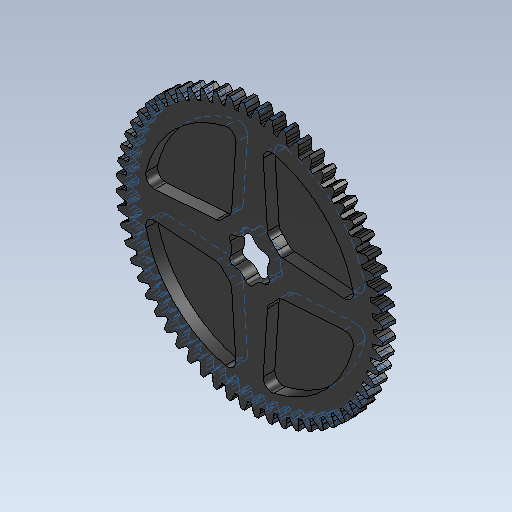
# Autodesk Inventor part: m1z60
Saved by Autodesk Inventor 2020 (Build 240168000, 168)
## iProperties
Created: 2020-10-28
Part Number: m1z60
Material: ポリカーボネート、クリア
Document SubType Name: Modeling
Designer: AA19065
Density: 1.2 g/cm^3
Appearance: 光沢 - 黒
Mass: 5.9358 g
Surface Area: 74.7819 cm^2
Volume: 4.9465 cm^3
Author: AA19065
Autodesk Inventor part; units mm, degrees
(part 1 of 2)
ref_plane "YZ Plane" through (0, 0, 0) normal (1, 0, 0) x (0, 1, 0)
ref_plane "XZ Plane" through (0, 0, 0) normal (0, 1, 0) x (-1, 0, 0)
ref_plane "XY Plane" through (0, 0, 0) normal (0, 0, 1) x (1, 0, 0)
sketch "スケッチ1" plane through (0, 0, 0) normal (0, 0, 1) x (1, 0, 0)
  arc A0 (149.0364, 134.2758) -> (148.8992, 133.7472) centre (155.551, 132.3028) ccw
  arc A1 (149.2947, 135.0135) -> (149.0364, 134.2758) centre (157.799, 131.622) ccw
  arc A2 (149.73, 135.9756) -> (149.2947, 135.0135) centre (160.0948, 130.7064) ccw
  arc A3 (145.9733, 134.1715) -> (145.8921, 133.6315) centre (152.6585, 132.8903) ccw
  arc A4 (146.1531, 134.9321) -> (145.9733, 134.1715) centre (154.9653, 132.4481) ccw
  arc A5 (146.4854, 135.9345) -> (146.1531, 134.9321) centre (157.3443, 131.7776) ccw
  arc A6 (142.9379, 133.7476) -> (142.9136, 133.202) centre (149.7204, 133.1722) ccw
  arc A7 (143.0372, 134.5228) -> (142.9379, 133.7476) centre (152.0608, 132.9736) ccw
  arc A8 (143.2629, 135.5544) -> (143.0372, 134.5228) centre (154.4968, 132.5553) ccw
  arc A9 (139.9634, 133.0087) -> (139.9963, 132.4636) centre (146.7689, 133.1454) ccw
  arc A10 (139.9811, 133.7901) -> (139.9634, 133.0087) centre (149.1173, 133.1925) ccw
  arc A11 (140.0978, 134.8396) -> (139.9811, 133.7901) centre (151.5836, 133.0312) ccw
  arc A12 (137.0825, 131.963) -> (137.1722, 131.4243) centre (143.8364, 132.8103) ccw
  arc A13 (137.0184, 132.7419) -> (137.0825, 131.963) centre (146.167, 133.1026) ccw
  arc A14 (137.0248, 133.7979) -> (137.0184, 132.7419) centre (148.6367, 133.2) ccw
  arc A15 (134.3267, 130.6218) -> (134.4721, 130.0954) centre (140.955, 132.1704) ccw
  arc A16 (134.1815, 131.3898) -> (134.3267, 130.6218) centre (143.2422, 132.7048) ccw
  arc A17 (134.0774, 132.4406) -> (134.1815, 131.3898) centre (145.6882, 133.0598) ccw
  arc A18 (131.7261, 128.9999) -> (131.9258, 128.4916) centre (138.1562, 131.2329) ccw
  arc A19 (131.5014, 129.7485) -> (131.7261, 128.9999) centre (140.3751, 132.0034) ccw
  arc A20 (131.2881, 130.7827) -> (131.5014, 129.7485) centre (142.7706, 132.6122) ccw
  arc A21 (129.3093, 127.1151) -> (129.561, 126.6305) centre (135.4708, 130.008) ccw
  arc A22 (129.0076, 127.8361) -> (129.3093, 127.1151) centre (137.597, 131.0062) ccw
  arc A23 (128.6874, 128.8424) -> (129.0076, 127.8361) centre (139.9157, 131.862) ccw
  arc A24 (127.1028, 124.988) -> (127.4038, 124.5323) centre (132.9281, 128.5091) ccw
  arc A25 (126.7274, 125.6735) -> (127.1028, 124.988) centre (134.9383, 129.7241) ccw
  arc A26 (126.3037, 126.6408) -> (126.7274, 125.6735) centre (137.1549, 130.8176) ccw
  arc A27 (125.1307, 122.6419) -> (125.4777, 122.2202) centre (130.5561, 126.7526) ccw
  arc A28 (124.6857, 123.2844) -> (125.1307, 122.6419) centre (132.4282, 128.1711) ccw
  arc A29 (124.1632, 124.2021) -> (124.6857, 123.2844) centre (134.5184, 129.4903) ccw
  arc A30 (123.4146, 120.1025) -> (123.8038, 119.7193) centre (128.3806, 124.7578) ccw
  arc A31 (122.9049, 120.695) -> (123.4146, 120.1025) centre (130.0942, 126.3642) ccw
  arc A32 (122.2894, 121.553) -> (122.9049, 120.695) centre (132.035, 127.8946) ccw
  arc A33 (121.9734, 117.3976) -> (122.4005, 117.0573) centre (126.4256, 122.5465) ccw
  arc A34 (121.4046, 117.9336) -> (121.9734, 117.3976) centre (127.9619, 124.3232) ccw
  arc A35 (120.7027, 118.7226) -> (121.4046, 117.9336) centre (129.7321, 126.0481) ccw
  arc A36 (120.8228, 114.5569) -> (121.2831, 114.2631) centre (124.7124, 120.143) ccw
  arc A37 (120.2011, 115.0305) -> (120.8228, 114.5569) centre (126.0546, 122.0705) ccw
  arc A38 (119.4206, 115.7418) -> (120.2011, 115.0305) centre (127.6348, 123.9711) ccw
  arc A39 (119.9755, 111.6115) -> (120.464, 111.3674) centre (123.2598, 117.5735) ccw
  arc A40 (119.3076, 112.0175) -> (119.9755, 111.6115) centre (124.3932, 119.6308) ccw
  arc A41 (118.457, 112.6433) -> (119.3076, 112.0175) centre (125.7661, 121.6861) ccw
  arc A42 (119.4406, 108.5937) -> (119.952, 108.4019) centre (122.0838, 114.8663) ccw
  arc A43 (118.734, 108.9276) -> (119.4406, 108.5937) centre (122.9959, 117.0308) ccw
  arc A44 (117.8227, 109.4611) -> (118.734, 108.9276) centre (124.1464, 119.2184) ccw
  arc A45 (119.2242, 105.5364) -> (119.7528, 105.3992) centre (121.1972, 112.051) ccw
  arc A46 (118.4865, 105.7947) -> (119.2242, 105.5364) centre (121.878, 114.299) ccw
  arc A47 (117.5244, 106.23) -> (118.4865, 105.7947) centre (122.7936, 116.5948) ccw
  arc A48 (119.3285, 102.4733) -> (119.8685, 102.3921) centre (120.6097, 109.1585) ccw
  arc A49 (118.5679, 102.6531) -> (119.3285, 102.4733) centre (121.0519, 111.4653) ccw
  arc A50 (117.5655, 102.9854) -> (118.5679, 102.6531) centre (121.7224, 113.8443) ccw
  arc A51 (119.7524, 99.4379) -> (120.298, 99.4136) centre (120.3278, 106.2204) ccw
  arc A52 (118.9772, 99.5372) -> (119.7524, 99.4379) centre (120.5264, 108.5608) ccw
  arc A53 (117.9456, 99.7629) -> (118.9772, 99.5372) centre (120.9447, 110.9968) ccw
  arc A54 (120.4913, 96.4634) -> (121.0364, 96.4963) centre (120.3546, 103.2689) ccw
  arc A55 (119.7099, 96.4811) -> (120.4913, 96.4634) centre (120.3075, 105.6173) ccw
  arc A56 (118.6604, 96.5978) -> (119.7099, 96.4811) centre (120.4688, 108.0836) ccw
  arc A57 (121.537, 93.5825) -> (122.0757, 93.6722) centre (120.6897, 100.3364) ccw
  arc A58 (120.7581, 93.5184) -> (121.537, 93.5825) centre (120.3974, 102.667) ccw
  arc A59 (119.7021, 93.5248) -> (120.7581, 93.5184) centre (120.3, 105.1367) ccw
  arc A60 (122.8782, 90.8267) -> (123.4046, 90.9721) centre (121.3296, 97.455) ccw
  arc A61 (122.1102, 90.6815) -> (122.8782, 90.8267) centre (120.7952, 99.7422) ccw
  arc A62 (121.0594, 90.5774) -> (122.1102, 90.6815) centre (120.4402, 102.1882) ccw
  arc A63 (124.5001, 88.2261) -> (125.0084, 88.4258) centre (122.2671, 94.6562) ccw
  arc A64 (123.7515, 88.0014) -> (124.5001, 88.2261) centre (121.4966, 96.8751) ccw
  arc A65 (122.7173, 87.7881) -> (123.7515, 88.0014) centre (120.8878, 99.2706) ccw
  arc A66 (126.3849, 85.8093) -> (126.8695, 86.061) centre (123.492, 91.9708) ccw
  arc A67 (125.6639, 85.5076) -> (126.3849, 85.8093) centre (122.4938, 94.097) ccw
  arc A68 (124.6576, 85.1874) -> (125.6639, 85.5076) centre (121.638, 96.4157) ccw
  arc A69 (128.512, 83.6028) -> (128.9677, 83.9038) centre (124.9909, 89.4281) ccw
  arc A70 (127.8265, 83.2274) -> (128.512, 83.6028) centre (123.7759, 91.4383) ccw
  arc A71 (126.8592, 82.8037) -> (127.8265, 83.2274) centre (122.6824, 93.6549) ccw
  arc A72 (130.8581, 81.6307) -> (131.2798, 81.9777) centre (126.7474, 87.0561) ccw
  arc A73 (130.2156, 81.1857) -> (130.8581, 81.6307) centre (125.3289, 88.9282) ccw
  arc A74 (129.2979, 80.6632) -> (130.2156, 81.1857) centre (124.0097, 91.0184) ccw
  arc A75 (133.3975, 79.9146) -> (133.7807, 80.3038) centre (128.7422, 84.8806) ccw
  arc A76 (132.805, 79.4049) -> (133.3975, 79.9146) centre (127.1358, 86.5942) ccw
  arc A77 (131.947, 78.7894) -> (132.805, 79.4049) centre (125.6054, 88.535) ccw
  arc A78 (136.1024, 78.4734) -> (136.4427, 78.9005) centre (130.9535, 82.9256) ccw
  arc A79 (135.5664, 77.9046) -> (136.1024, 78.4734) centre (129.1768, 84.4619) ccw
  arc A80 (134.7774, 77.2027) -> (135.5664, 77.9046) centre (127.4519, 86.2321) ccw
  arc A81 (138.9431, 77.3228) -> (139.2369, 77.7831) centre (133.357, 81.2124) ccw
  arc A82 (138.4695, 76.7011) -> (138.9431, 77.3228) centre (131.4295, 82.5546) ccw
  arc A83 (137.7582, 75.9206) -> (138.4695, 76.7011) centre (129.529, 84.1348) ccw
  arc A84 (141.8885, 76.4755) -> (142.1326, 76.964) centre (135.9265, 79.7598) ccw
  arc A85 (141.4825, 75.8076) -> (141.8885, 76.4755) centre (133.8692, 80.8932) ccw
  arc A86 (140.8567, 74.957) -> (141.4825, 75.8076) centre (131.8139, 82.2661) ccw
  arc A87 (144.9063, 75.9406) -> (145.0981, 76.452) centre (138.6337, 78.5838) ccw
  arc A88 (144.5724, 75.234) -> (144.9063, 75.9406) centre (136.4692, 79.4959) ccw
  arc A89 (144.0389, 74.3227) -> (144.5724, 75.234) centre (134.2816, 80.6464) ccw
  arc A90 (147.9636, 75.7242) -> (148.1008, 76.2528) centre (141.449, 77.6972) ccw
  arc A91 (147.7053, 74.9865) -> (147.9636, 75.7242) centre (139.201, 78.378) ccw
  arc A92 (147.27, 74.0244) -> (147.7053, 74.9865) centre (136.9052, 79.2936) ccw
  arc A93 (151.0267, 75.8285) -> (151.1079, 76.3685) centre (144.3415, 77.1097) ccw
  arc A94 (150.8469, 75.0679) -> (151.0267, 75.8285) centre (142.0347, 77.5519) ccw
  arc A95 (150.5146, 74.0655) -> (150.8469, 75.0679) centre (139.6557, 78.2224) ccw
  arc A96 (154.0621, 76.2524) -> (154.0864, 76.798) centre (147.2796, 76.8278) ccw
  arc A97 (153.9628, 75.4772) -> (154.0621, 76.2524) centre (144.9392, 77.0264) ccw
  arc A98 (153.7371, 74.4456) -> (153.9628, 75.4772) centre (142.5032, 77.4447) ccw
  arc A99 (157.0366, 76.9913) -> (157.0037, 77.5364) centre (150.2311, 76.8546) ccw
  arc A100 (157.0189, 76.2099) -> (157.0366, 76.9913) centre (147.8827, 76.8075) ccw
  arc A101 (156.9022, 75.1604) -> (157.0189, 76.2099) centre (145.4164, 76.9688) ccw
  arc A102 (159.9175, 78.037) -> (159.8278, 78.5757) centre (153.1636, 77.1897) ccw
  arc A103 (159.9816, 77.2581) -> (159.9175, 78.037) centre (150.833, 76.8974) ccw
  arc A104 (159.9752, 76.2021) -> (159.9816, 77.2581) centre (148.3633, 76.8) ccw
  arc A105 (162.6733, 79.3782) -> (162.5279, 79.9046) centre (156.045, 77.8296) ccw
  arc A106 (162.8185, 78.6102) -> (162.6733, 79.3782) centre (153.7578, 77.2952) ccw
  arc A107 (162.9226, 77.5594) -> (162.8185, 78.6102) centre (151.3118, 76.9402) ccw
  arc A108 (165.2739, 81.0001) -> (165.0742, 81.5084) centre (158.8438, 78.7671) ccw
  arc A109 (165.4986, 80.2515) -> (165.2739, 81.0001) centre (156.6249, 77.9966) ccw
  arc A110 (165.7119, 79.2173) -> (165.4986, 80.2515) centre (154.2294, 77.3878) ccw
  arc A111 (167.6907, 82.8849) -> (167.439, 83.3695) centre (161.5292, 79.992) ccw
  arc A112 (167.9924, 82.1639) -> (167.6907, 82.8849) centre (159.403, 78.9938) ccw
  arc A113 (168.3126, 81.1576) -> (167.9924, 82.1639) centre (157.0843, 78.138) ccw
  arc A114 (169.8972, 85.012) -> (169.5962, 85.4677) centre (164.0719, 81.4909) ccw
  arc A115 (170.2726, 84.3265) -> (169.8972, 85.012) centre (162.0617, 80.2759) ccw
  arc A116 (170.6963, 83.3592) -> (170.2726, 84.3265) centre (159.8451, 79.1824) ccw
  arc A117 (171.8693, 87.3581) -> (171.5223, 87.7798) centre (166.4439, 83.2474) ccw
  arc A118 (172.3143, 86.7156) -> (171.8693, 87.3581) centre (164.5718, 81.8289) ccw
  arc A119 (172.8368, 85.7979) -> (172.3143, 86.7156) centre (162.4816, 80.5097) ccw
  arc A120 (173.5854, 89.8975) -> (173.1962, 90.2807) centre (168.6194, 85.2422) ccw
  arc A121 (174.0951, 89.305) -> (173.5854, 89.8975) centre (166.9058, 83.6358) ccw
  arc A122 (174.7106, 88.447) -> (174.0951, 89.305) centre (164.965, 82.1054) ccw
  arc A123 (175.0266, 92.6024) -> (174.5995, 92.9427) centre (170.5744, 87.4535) ccw
  arc A124 (175.5954, 92.0664) -> (175.0266, 92.6024) centre (169.0381, 85.6768) ccw
  arc A125 (176.2973, 91.2774) -> (175.5954, 92.0664) centre (167.2679, 83.9519) ccw
  arc A126 (176.1772, 95.4431) -> (175.7169, 95.7369) centre (172.2876, 89.857) ccw
  arc A127 (176.7989, 94.9695) -> (176.1772, 95.4431) centre (170.9454, 87.9295) ccw
  arc A128 (177.5794, 94.2582) -> (176.7989, 94.9695) centre (169.3652, 86.029) ccw
  arc A129 (177.0245, 98.3885) -> (176.536, 98.6326) centre (173.7402, 92.4265) ccw
  arc A130 (177.6924, 97.9825) -> (177.0245, 98.3885) centre (172.6068, 90.3692) ccw
  arc A131 (178.543, 97.3567) -> (177.6924, 97.9825) centre (171.2339, 88.3139) ccw
  arc A132 (177.5594, 101.4063) -> (177.048, 101.5981) centre (174.9162, 95.1337) ccw
  arc A133 (178.266, 101.0724) -> (177.5594, 101.4063) centre (174.0041, 92.9692) ccw
  arc A134 (179.1773, 100.5389) -> (178.266, 101.0724) centre (172.8536, 90.7816) ccw
  arc A135 (177.7758, 104.4636) -> (177.2472, 104.6008) centre (175.8028, 97.949) ccw
  arc A136 (178.5135, 104.2053) -> (177.7758, 104.4636) centre (175.122, 95.701) ccw
  arc A137 (179.4756, 103.77) -> (178.5135, 104.2053) centre (174.2064, 93.4052) ccw
  arc A138 (177.6715, 107.5267) -> (177.1315, 107.6079) centre (176.3903, 100.8415) ccw
  arc A139 (178.4321, 107.3469) -> (177.6715, 107.5267) centre (175.9481, 98.5347) ccw
  arc A140 (179.4345, 107.0146) -> (178.4321, 107.3469) centre (175.2776, 96.1557) ccw
  arc A141 (177.2476, 110.5621) -> (176.702, 110.5864) centre (176.6722, 103.7796) ccw
  arc A142 (178.0228, 110.4628) -> (177.2476, 110.5621) centre (176.4736, 101.4392) ccw
  arc A143 (179.0544, 110.2371) -> (178.0228, 110.4628) centre (176.0553, 99.0032) ccw
  arc A144 (176.5087, 113.5366) -> (175.9636, 113.5037) centre (176.6454, 106.7311) ccw
  arc A145 (177.2901, 113.5189) -> (176.5087, 113.5366) centre (176.6925, 104.3827) ccw
  arc A146 (178.3396, 113.4022) -> (177.2901, 113.5189) centre (176.5312, 101.9164) ccw
  arc A147 (175.463, 116.4175) -> (174.9243, 116.3278) centre (176.3103, 109.6636) ccw
  arc A148 (176.2419, 116.4816) -> (175.463, 116.4175) centre (176.6026, 107.333) ccw
  arc A149 (177.2979, 116.4752) -> (176.2419, 116.4816) centre (176.7, 104.8633) ccw
  arc A150 (174.1218, 119.1734) -> (173.5954, 119.0279) centre (175.6704, 112.545) ccw
  arc A151 (174.8898, 119.3185) -> (174.1218, 119.1734) centre (176.2048, 110.2578) ccw
  arc A152 (175.9406, 119.4226) -> (174.8898, 119.3185) centre (176.5598, 107.8118) ccw
  arc A153 (172.4999, 121.7739) -> (171.9916, 121.5742) centre (174.7329, 115.3438) ccw
  arc A154 (173.2485, 121.9986) -> (172.4999, 121.7739) centre (175.5034, 113.1249) ccw
  arc A155 (174.2827, 122.2119) -> (173.2485, 121.9986) centre (176.1122, 110.7294) ccw
  arc A156 (170.6151, 124.1907) -> (170.1305, 123.939) centre (173.508, 118.0292) ccw
  arc A157 (171.3361, 124.4924) -> (170.6151, 124.1907) centre (174.5062, 115.903) ccw
  arc A158 (172.3424, 124.8126) -> (171.3361, 124.4924) centre (175.362, 113.5843) ccw
  arc A159 (168.488, 126.3972) -> (168.0323, 126.0962) centre (172.0091, 120.5719) ccw
  arc A160 (169.1735, 126.7726) -> (168.488, 126.3972) centre (173.2241, 118.5617) ccw
  arc A161 (170.1408, 127.1963) -> (169.1735, 126.7726) centre (174.3176, 116.3451) ccw
  arc A162 (166.1419, 128.3693) -> (165.7202, 128.0223) centre (170.2526, 122.9439) ccw
  arc A163 (166.7844, 128.8143) -> (166.1419, 128.3693) centre (171.6711, 121.0718) ccw
  arc A164 (167.7021, 129.3368) -> (166.7844, 128.8143) centre (172.9903, 118.9816) ccw
  arc A165 (163.6025, 130.0854) -> (163.2193, 129.6962) centre (168.2578, 125.1194) ccw
  arc A166 (164.195, 130.5951) -> (163.6025, 130.0854) centre (169.8642, 123.4058) ccw
  arc A167 (165.053, 131.2106) -> (164.195, 130.5951) centre (171.3946, 121.465) ccw
  arc A168 (160.8976, 131.5266) -> (160.5573, 131.0995) centre (166.0465, 127.0744) ccw
  arc A169 (161.4336, 132.0954) -> (160.8976, 131.5266) centre (167.8232, 125.5381) ccw
  arc A170 (162.2226, 132.7973) -> (161.4336, 132.0954) centre (169.5481, 123.7679) ccw
  arc A171 (158.0569, 132.6772) -> (157.7631, 132.2169) centre (163.643, 128.7876) ccw
  arc A172 (158.5305, 133.2989) -> (158.0569, 132.6772) centre (165.5705, 127.4454) ccw
  arc A173 (159.2418, 134.0794) -> (158.5305, 133.2989) centre (167.471, 125.8652) ccw
  arc A174 (155.1115, 133.5245) -> (154.8674, 133.036) centre (161.0735, 130.2402) ccw
  arc A175 (155.5175, 134.1924) -> (155.1115, 133.5245) centre (163.1308, 129.1068) ccw
  arc A176 (156.1433, 135.043) -> (155.5175, 134.1924) centre (165.1861, 127.7339) ccw
  arc A177 (152.0936, 134.0594) -> (151.9019, 133.548) centre (158.3663, 131.4162) ccw
  arc A178 (152.4276, 134.766) -> (152.0936, 134.0594) centre (160.5308, 130.5041) ccw
  arc A179 (152.9611, 135.6773) -> (152.4276, 134.766) centre (162.7184, 129.3536) ccw
  arc A180 (148.1008, 133.7472) -> (147.9636, 134.2758) centre (141.449, 132.3028) ccw
  arc A181 (147.9636, 134.2758) -> (147.7053, 135.0135) centre (139.201, 131.622) ccw
  arc A182 (147.7053, 135.0135) -> (147.27, 135.9756) centre (136.9052, 130.7064) ccw
  arc A183 (145.0981, 133.548) -> (144.9063, 134.0594) centre (138.6337, 131.4162) ccw
  arc A184 (144.9063, 134.0594) -> (144.5724, 134.766) centre (136.4692, 130.5041) ccw
  arc A185 (144.5724, 134.766) -> (144.0389, 135.6773) centre (134.2816, 129.3536) ccw
  arc A186 (142.1326, 133.036) -> (141.8885, 133.5245) centre (135.9265, 130.2402) ccw
  arc A187 (141.8885, 133.5245) -> (141.4825, 134.1924) centre (133.8692, 129.1068) ccw
  arc A188 (141.4825, 134.1924) -> (140.8567, 135.043) centre (131.8139, 127.7339) ccw
  arc A189 (139.2369, 132.2169) -> (138.9431, 132.6772) centre (133.357, 128.7876) ccw
  arc A190 (138.9431, 132.6772) -> (138.4695, 133.2989) centre (131.4295, 127.4454) ccw
  arc A191 (138.4695, 133.2989) -> (137.7582, 134.0794) centre (129.529, 125.8652) ccw
  arc A192 (136.4427, 131.0995) -> (136.1024, 131.5266) centre (130.9535, 127.0744) ccw
  arc A193 (136.1024, 131.5266) -> (135.5664, 132.0954) centre (129.1768, 125.5381) ccw
  arc A194 (135.5664, 132.0954) -> (134.7774, 132.7973) centre (127.4519, 123.7679) ccw
  arc A195 (133.7807, 129.6962) -> (133.3975, 130.0854) centre (128.7422, 125.1194) ccw
  arc A196 (133.3975, 130.0854) -> (132.805, 130.5951) centre (127.1358, 123.4058) ccw
  arc A197 (132.805, 130.5951) -> (131.947, 131.2106) centre (125.6054, 121.465) ccw
  arc A198 (131.2798, 128.0223) -> (130.8581, 128.3693) centre (126.7474, 122.9439) ccw
  arc A199 (130.8581, 128.3693) -> (130.2156, 128.8143) centre (125.3289, 121.0718) ccw
  arc A200 (130.2156, 128.8143) -> (129.2979, 129.3368) centre (124.0097, 118.9816) ccw
  arc A201 (128.9677, 126.0962) -> (128.512, 126.3972) centre (124.9909, 120.5719) ccw
  arc A202 (128.512, 126.3972) -> (127.8265, 126.7726) centre (123.7759, 118.5617) ccw
  arc A203 (127.8265, 126.7726) -> (126.8592, 127.1963) centre (122.6824, 116.3451) ccw
  arc A204 (126.8695, 123.939) -> (126.3849, 124.1907) centre (123.492, 118.0292) ccw
  arc A205 (126.3849, 124.1907) -> (125.6639, 124.4924) centre (122.4938, 115.903) ccw
  arc A206 (125.6639, 124.4924) -> (124.6576, 124.8126) centre (121.638, 113.5843) ccw
  arc A207 (125.0084, 121.5742) -> (124.5001, 121.7739) centre (122.2671, 115.3438) ccw
  arc A208 (124.5001, 121.7739) -> (123.7515, 121.9986) centre (121.4966, 113.1249) ccw
  arc A209 (123.7515, 121.9986) -> (122.7173, 122.2119) centre (120.8878, 110.7294) ccw
  arc A210 (123.4046, 119.0279) -> (122.8782, 119.1733) centre (121.3296, 112.545) ccw
  arc A211 (122.8782, 119.1733) -> (122.1102, 119.3185) centre (120.7952, 110.2578) ccw
  arc A212 (122.1102, 119.3185) -> (121.0594, 119.4226) centre (120.4402, 107.8118) ccw
  arc A213 (122.0757, 116.3278) -> (121.537, 116.4175) centre (120.6897, 109.6636) ccw
  arc A214 (121.537, 116.4175) -> (120.7581, 116.4816) centre (120.3974, 107.333) ccw
  arc A215 (120.7581, 116.4816) -> (119.7021, 116.4752) centre (120.3, 104.8633) ccw
  arc A216 (121.0364, 113.5037) -> (120.4913, 113.5366) centre (120.3546, 106.7311) ccw
  arc A217 (120.4913, 113.5366) -> (119.7099, 113.5189) centre (120.3075, 104.3827) ccw
  arc A218 (119.7099, 113.5189) -> (118.6604, 113.4022) centre (120.4688, 101.9164) ccw
  arc A219 (120.298, 110.5864) -> (119.7524, 110.5621) centre (120.3278, 103.7796) ccw
  arc A220 (119.7524, 110.5621) -> (118.9772, 110.4628) centre (120.5264, 101.4392) ccw
  arc A221 (118.9772, 110.4628) -> (117.9456, 110.2371) centre (120.9447, 99.0032) ccw
  arc A222 (119.8685, 107.6079) -> (119.3285, 107.5267) centre (120.6097, 100.8415) ccw
  arc A223 (119.3285, 107.5267) -> (118.5679, 107.3469) centre (121.0519, 98.5347) ccw
  arc A224 (118.5679, 107.3469) -> (117.5655, 107.0146) centre (121.7224, 96.1557) ccw
  arc A225 (119.7528, 104.6008) -> (119.2242, 104.4636) centre (121.1972, 97.949) ccw
  arc A226 (119.2242, 104.4636) -> (118.4865, 104.2053) centre (121.878, 95.701) ccw
  arc A227 (118.4865, 104.2053) -> (117.5244, 103.77) centre (122.7936, 93.4052) ccw
  arc A228 (119.952, 101.5981) -> (119.4406, 101.4063) centre (122.0838, 95.1337) ccw
  arc A229 (119.4406, 101.4063) -> (118.734, 101.0724) centre (122.9959, 92.9692) ccw
  arc A230 (118.734, 101.0724) -> (117.8227, 100.5389) centre (124.1464, 90.7816) ccw
  arc A231 (120.464, 98.6326) -> (119.9755, 98.3885) centre (123.2598, 92.4265) ccw
  arc A232 (119.9755, 98.3885) -> (119.3076, 97.9825) centre (124.3932, 90.3692) ccw
  arc A233 (119.3076, 97.9825) -> (118.457, 97.3567) centre (125.7661, 88.3139) ccw
  arc A234 (121.2831, 95.7369) -> (120.8228, 95.4431) centre (124.7124, 89.857) ccw
  arc A235 (120.8228, 95.4431) -> (120.2011, 94.9695) centre (126.0546, 87.9295) ccw
  arc A236 (120.2011, 94.9695) -> (119.4206, 94.2582) centre (127.6348, 86.0289) ccw
  arc A237 (122.4005, 92.9427) -> (121.9734, 92.6024) centre (126.4256, 87.4535) ccw
  arc A238 (121.9734, 92.6024) -> (121.4046, 92.0664) centre (127.9619, 85.6768) ccw
  arc A239 (121.4046, 92.0664) -> (120.7027, 91.2774) centre (129.7321, 83.9519) ccw
  arc A240 (123.8038, 90.2807) -> (123.4146, 89.8975) centre (128.3806, 85.2422) ccw
  arc A241 (123.4146, 89.8975) -> (122.9049, 89.305) centre (130.0942, 83.6358) ccw
  arc A242 (122.9049, 89.305) -> (122.2894, 88.447) centre (132.035, 82.1054) ccw
  arc A243 (125.4777, 87.7798) -> (125.1307, 87.3581) centre (130.5561, 83.2474) ccw
  arc A244 (125.1307, 87.3581) -> (124.6857, 86.7156) centre (132.4282, 81.8289) ccw
  arc A245 (124.6857, 86.7156) -> (124.1632, 85.7979) centre (134.5184, 80.5097) ccw
  arc A246 (127.4038, 85.4677) -> (127.1028, 85.012) centre (132.9281, 81.4909) ccw
  arc A247 (127.1028, 85.012) -> (126.7274, 84.3265) centre (134.9383, 80.2759) ccw
  arc A248 (126.7274, 84.3265) -> (126.3037, 83.3592) centre (137.1549, 79.1824) ccw
  arc A249 (129.561, 83.3695) -> (129.3093, 82.8849) centre (135.4708, 79.992) ccw
  arc A250 (129.3093, 82.8849) -> (129.0076, 82.1639) centre (137.597, 78.9938) ccw
  arc A251 (129.0076, 82.1639) -> (128.6874, 81.1576) centre (139.9157, 78.138) ccw
  arc A252 (131.9258, 81.5084) -> (131.7261, 81.0001) centre (138.1562, 78.7671) ccw
  arc A253 (131.7261, 81.0001) -> (131.5014, 80.2515) centre (140.3751, 77.9966) ccw
  arc A254 (131.5014, 80.2515) -> (131.2881, 79.2173) centre (142.7706, 77.3878) ccw
  arc A255 (134.4721, 79.9046) -> (134.3267, 79.3782) centre (140.955, 77.8296) ccw
  arc A256 (134.3267, 79.3782) -> (134.1815, 78.6102) centre (143.2422, 77.2952) ccw
  arc A257 (134.1815, 78.6102) -> (134.0774, 77.5594) centre (145.6882, 76.9402) ccw
  arc A258 (137.1722, 78.5757) -> (137.0825, 78.037) centre (143.8364, 77.1897) ccw
  arc A259 (137.0825, 78.037) -> (137.0184, 77.2581) centre (146.167, 76.8974) ccw
  arc A260 (137.0184, 77.2581) -> (137.0248, 76.2021) centre (148.6367, 76.8) ccw
  arc A261 (139.9963, 77.5364) -> (139.9634, 76.9913) centre (146.7689, 76.8546) ccw
  arc A262 (139.9634, 76.9913) -> (139.9811, 76.2099) centre (149.1173, 76.8075) ccw
  arc A263 (139.9811, 76.2099) -> (140.0978, 75.1604) centre (151.5836, 76.9688) ccw
  arc A264 (142.9136, 76.798) -> (142.9379, 76.2524) centre (149.7204, 76.8278) ccw
  arc A265 (142.9379, 76.2524) -> (143.0372, 75.4772) centre (152.0608, 77.0264) ccw
  arc A266 (143.0372, 75.4772) -> (143.2629, 74.4456) centre (154.4968, 77.4447) ccw
  arc A267 (145.8921, 76.3685) -> (145.9733, 75.8285) centre (152.6585, 77.1097) ccw
  arc A268 (145.9733, 75.8285) -> (146.1531, 75.0679) centre (154.9653, 77.5519) ccw
  arc A269 (146.1531, 75.0679) -> (146.4854, 74.0655) centre (157.3443, 78.2224) ccw
  arc A270 (148.8992, 76.2528) -> (149.0364, 75.7242) centre (155.551, 77.6972) ccw
  arc A271 (149.0364, 75.7242) -> (149.2947, 74.9865) centre (157.799, 78.378) ccw
  arc A272 (149.2947, 74.9865) -> (149.73, 74.0244) centre (160.0948, 79.2936) ccw
  arc A273 (151.9019, 76.452) -> (152.0936, 75.9406) centre (158.3663, 78.5838) ccw
  arc A274 (152.0936, 75.9406) -> (152.4276, 75.234) centre (160.5308, 79.4959) ccw
  arc A275 (152.4276, 75.234) -> (152.9611, 74.3227) centre (162.7184, 80.6464) ccw
  arc A276 (154.8674, 76.964) -> (155.1115, 76.4755) centre (161.0735, 79.7598) ccw
  arc A277 (155.1115, 76.4755) -> (155.5175, 75.8076) centre (163.1308, 80.8932) ccw
  arc A278 (155.5175, 75.8076) -> (156.1433, 74.957) centre (165.1861, 82.2661) ccw
  arc A279 (157.7631, 77.7831) -> (158.0569, 77.3228) centre (163.643, 81.2124) ccw
  arc A280 (158.0569, 77.3228) -> (158.5305, 76.7011) centre (165.5705, 82.5546) ccw
  arc A281 (158.5305, 76.7011) -> (159.2418, 75.9206) centre (167.471, 84.1348) ccw
  arc A282 (160.5573, 78.9005) -> (160.8976, 78.4734) centre (166.0465, 82.9256) ccw
  arc A283 (160.8976, 78.4734) -> (161.4336, 77.9046) centre (167.8232, 84.4619) ccw
  arc A284 (161.4336, 77.9046) -> (162.2226, 77.2027) centre (169.5481, 86.2321) ccw
  arc A285 (163.2193, 80.3038) -> (163.6025, 79.9146) centre (168.2578, 84.8806) ccw
  arc A286 (163.6025, 79.9146) -> (164.195, 79.4049) centre (169.8642, 86.5942) ccw
  arc A287 (164.195, 79.4049) -> (165.053, 78.7894) centre (171.3946, 88.535) ccw
  arc A288 (165.7202, 81.9777) -> (166.1419, 81.6307) centre (170.2526, 87.0561) ccw
  arc A289 (166.1419, 81.6307) -> (166.7844, 81.1857) centre (171.6711, 88.9282) ccw
  arc A290 (166.7844, 81.1857) -> (167.7021, 80.6632) centre (172.9903, 91.0184) ccw
  arc A291 (168.0323, 83.9038) -> (168.488, 83.6028) centre (172.0091, 89.4281) ccw
  arc A292 (168.488, 83.6028) -> (169.1735, 83.2274) centre (173.2241, 91.4383) ccw
  arc A293 (169.1735, 83.2274) -> (170.1408, 82.8037) centre (174.3176, 93.6549) ccw
  arc A294 (170.1305, 86.061) -> (170.6151, 85.8093) centre (173.508, 91.9708) ccw
  arc A295 (170.6151, 85.8093) -> (171.3361, 85.5076) centre (174.5062, 94.097) ccw
  arc A296 (171.3361, 85.5076) -> (172.3424, 85.1874) centre (175.362, 96.4157) ccw
  arc A297 (171.9916, 88.4258) -> (172.4999, 88.2261) centre (174.7329, 94.6562) ccw
  arc A298 (172.4999, 88.2261) -> (173.2485, 88.0014) centre (175.5034, 96.8751) ccw
  arc A299 (173.2485, 88.0014) -> (174.2827, 87.7881) centre (176.1122, 99.2706) ccw
  arc A300 (173.5954, 90.9721) -> (174.1218, 90.8266) centre (175.6704, 97.455) ccw
  arc A301 (174.1218, 90.8266) -> (174.8898, 90.6815) centre (176.2048, 99.7422) ccw
  arc A302 (174.8898, 90.6815) -> (175.9406, 90.5774) centre (176.5598, 102.1882) ccw
  arc A303 (174.9243, 93.6722) -> (175.463, 93.5825) centre (176.3103, 100.3364) ccw
  arc A304 (175.463, 93.5825) -> (176.2419, 93.5184) centre (176.6026, 102.667) ccw
  arc A305 (176.2419, 93.5184) -> (177.2979, 93.5248) centre (176.7, 105.1367) ccw
  arc A306 (175.9636, 96.4963) -> (176.5087, 96.4634) centre (176.6454, 103.2689) ccw
  arc A307 (176.5087, 96.4634) -> (177.2901, 96.4811) centre (176.6925, 105.6173) ccw
  arc A308 (177.2901, 96.4811) -> (178.3396, 96.5978) centre (176.5312, 108.0836) ccw
  arc A309 (176.702, 99.4136) -> (177.2476, 99.4379) centre (176.6722, 106.2204) ccw
  arc A310 (177.2476, 99.4379) -> (178.0228, 99.5372) centre (176.4736, 108.5608) ccw
  arc A311 (178.0228, 99.5372) -> (179.0544, 99.7629) centre (176.0553, 110.9968) ccw
  arc A312 (177.1315, 102.3921) -> (177.6715, 102.4733) centre (176.3903, 109.1585) ccw
  arc A313 (177.6715, 102.4733) -> (178.4321, 102.6531) centre (175.9481, 111.4653) ccw
  arc A314 (178.4321, 102.6531) -> (179.4345, 102.9854) centre (175.2776, 113.8443) ccw
  arc A315 (177.2472, 105.3992) -> (177.7758, 105.5364) centre (175.8028, 112.051) ccw
  arc A316 (177.7758, 105.5364) -> (178.5135, 105.7947) centre (175.122, 114.299) ccw
  arc A317 (178.5135, 105.7947) -> (179.4756, 106.23) centre (174.2064, 116.5948) ccw
  arc A318 (177.048, 108.4019) -> (177.5594, 108.5937) centre (174.9162, 114.8663) ccw
  arc A319 (177.5594, 108.5937) -> (178.266, 108.9276) centre (174.0041, 117.0308) ccw
  arc A320 (178.266, 108.9276) -> (179.1773, 109.4611) centre (172.8536, 119.2184) ccw
  arc A321 (176.536, 111.3674) -> (177.0245, 111.6115) centre (173.7402, 117.5735) ccw
  arc A322 (177.0245, 111.6115) -> (177.6924, 112.0175) centre (172.6068, 119.6308) ccw
  arc A323 (177.6924, 112.0175) -> (178.543, 112.6433) centre (171.2339, 121.6861) ccw
  arc A324 (175.7169, 114.2631) -> (176.1772, 114.5569) centre (172.2876, 120.143) ccw
  arc A325 (176.1772, 114.5569) -> (176.7989, 115.0305) centre (170.9454, 122.0705) ccw
  arc A326 (176.7989, 115.0305) -> (177.5794, 115.7418) centre (169.3652, 123.971) ccw
  arc A327 (174.5995, 117.0573) -> (175.0266, 117.3976) centre (170.5744, 122.5465) ccw
  arc A328 (175.0266, 117.3976) -> (175.5954, 117.9336) centre (169.0381, 124.3232) ccw
  arc A329 (175.5954, 117.9336) -> (176.2973, 118.7226) centre (167.2679, 126.0481) ccw
  arc A330 (173.1962, 119.7193) -> (173.5854, 120.1025) centre (168.6194, 124.7578) ccw
  arc A331 (173.5854, 120.1025) -> (174.0951, 120.695) centre (166.9058, 126.3642) ccw
  arc A332 (174.0951, 120.695) -> (174.7106, 121.553) centre (164.965, 127.8946) ccw
  arc A333 (171.5223, 122.2202) -> (171.8693, 122.6419) centre (166.4439, 126.7526) ccw
  arc A334 (171.8693, 122.6419) -> (172.3143, 123.2844) centre (164.5718, 128.1711) ccw
  arc A335 (172.3143, 123.2844) -> (172.8368, 124.2021) centre (162.4816, 129.4903) ccw
  arc A336 (169.5962, 124.5323) -> (169.8972, 124.988) centre (164.0719, 128.5091) ccw
  arc A337 (169.8972, 124.988) -> (170.2726, 125.6735) centre (162.0617, 129.7241) ccw
  arc A338 (170.2726, 125.6735) -> (170.6963, 126.6408) centre (159.8451, 130.8176) ccw
  arc A339 (167.439, 126.6305) -> (167.6907, 127.1151) centre (161.5292, 130.008) ccw
  arc A340 (167.6907, 127.1151) -> (167.9924, 127.8361) centre (159.403, 131.0062) ccw
  arc A341 (167.9924, 127.8361) -> (168.3126, 128.8424) centre (157.0843, 131.862) ccw
  arc A342 (165.0742, 128.4916) -> (165.2739, 128.9999) centre (158.8438, 131.2329) ccw
  arc A343 (165.2739, 128.9999) -> (165.4986, 129.7485) centre (156.6249, 132.0034) ccw
  arc A344 (165.4986, 129.7485) -> (165.7119, 130.7827) centre (154.2294, 132.6122) ccw
  arc A345 (162.5279, 130.0954) -> (162.6733, 130.6218) centre (156.045, 132.1704) ccw
  arc A346 (162.6733, 130.6218) -> (162.8185, 131.3898) centre (153.7578, 132.7048) ccw
  arc A347 (162.8185, 131.3898) -> (162.9226, 132.4406) centre (151.3118, 133.0598) ccw
  arc A348 (159.8278, 131.4243) -> (159.9175, 131.963) centre (153.1636, 132.8103) ccw
  arc A349 (159.9175, 131.963) -> (159.9816, 132.7419) centre (150.833, 133.1026) ccw
  arc A350 (159.9816, 132.7419) -> (159.9752, 133.7979) centre (148.3633, 133.2) ccw
  arc A351 (157.0037, 132.4636) -> (157.0366, 133.0087) centre (150.2311, 133.1454) ccw
  arc A352 (157.0366, 133.0087) -> (157.0189, 133.7901) centre (147.8827, 133.1925) ccw
  arc A353 (157.0189, 133.7901) -> (156.9022, 134.8396) centre (145.4164, 133.0312) ccw
  arc A354 (154.0864, 133.202) -> (154.0621, 133.7476) centre (147.2796, 133.1722) ccw
  arc A355 (154.0621, 133.7476) -> (153.9628, 134.5228) centre (144.9392, 132.9736) ccw
  arc A356 (153.9628, 134.5228) -> (153.7371, 135.5544) centre (142.5032, 132.5553) ccw
  arc A357 (151.1079, 133.6315) -> (151.0267, 134.1715) centre (144.3415, 132.8903) ccw
  arc A358 (151.0267, 134.1715) -> (150.8469, 134.9321) centre (142.0347, 132.4481) ccw
  arc A359 (150.8469, 134.9321) -> (150.5146, 135.9345) centre (139.6557, 131.7776) ccw
  arc A360 (148.8992, 133.7472) -> (148.1008, 133.7472) centre (148.5, 105) ccw
  arc A361 (145.8921, 133.6315) -> (145.0981, 133.548) centre (148.5, 105) ccw
  arc A362 (142.9136, 133.202) -> (142.1326, 133.036) centre (148.5, 105) ccw
  arc A363 (139.9963, 132.4636) -> (139.2369, 132.2169) centre (148.5, 105) ccw
  arc A364 (137.1722, 131.4243) -> (136.4427, 131.0995) centre (148.5, 105) ccw
  arc A365 (134.4721, 130.0954) -> (133.7807, 129.6962) centre (148.5, 105) ccw
  arc A366 (131.9258, 128.4916) -> (131.2798, 128.0223) centre (148.5, 105) ccw
  arc A367 (129.561, 126.6305) -> (128.9677, 126.0962) centre (148.5, 105) ccw
  arc A368 (127.4038, 124.5323) -> (126.8695, 123.939) centre (148.5, 105) ccw
  arc A369 (125.4777, 122.2202) -> (125.0084, 121.5742) centre (148.5, 105) ccw
  arc A370 (123.8038, 119.7193) -> (123.4046, 119.0279) centre (148.5, 105) ccw
  arc A371 (122.4005, 117.0573) -> (122.0757, 116.3278) centre (148.5, 105) ccw
  arc A372 (121.2831, 114.2631) -> (121.0364, 113.5037) centre (148.5, 105) ccw
  arc A373 (120.464, 111.3674) -> (120.298, 110.5864) centre (148.5, 105) ccw
  arc A374 (119.952, 108.4019) -> (119.8685, 107.6079) centre (148.5, 105) ccw
  arc A375 (119.7528, 105.3992) -> (119.7528, 104.6008) centre (148.5, 105) ccw
  arc A376 (119.8685, 102.3921) -> (119.952, 101.5981) centre (148.5, 105) ccw
  arc A377 (120.298, 99.4136) -> (120.464, 98.6326) centre (148.5, 105) ccw
  arc A378 (121.0364, 96.4963) -> (121.2831, 95.7369) centre (148.5, 105) ccw
  arc A379 (122.0757, 93.6722) -> (122.4005, 92.9427) centre (148.5, 105) ccw
  arc A380 (123.4046, 90.9721) -> (123.8038, 90.2807) centre (148.5, 105) ccw
  arc A381 (125.0084, 88.4258) -> (125.4777, 87.7798) centre (148.5, 105) ccw
  arc A382 (126.8695, 86.061) -> (127.4038, 85.4677) centre (148.5, 105) ccw
  arc A383 (128.9677, 83.9038) -> (129.561, 83.3695) centre (148.5, 105) ccw
  arc A384 (131.2798, 81.9777) -> (131.9258, 81.5084) centre (148.5, 105) ccw
  arc A385 (133.7807, 80.3038) -> (134.4721, 79.9046) centre (148.5, 105) ccw
  arc A386 (136.4427, 78.9005) -> (137.1722, 78.5757) centre (148.5, 105) ccw
  arc A387 (139.2369, 77.7831) -> (139.9963, 77.5364) centre (148.5, 105) ccw
  arc A388 (142.1326, 76.964) -> (142.9136, 76.798) centre (148.5, 105) ccw
  arc A389 (145.0981, 76.452) -> (145.8921, 76.3685) centre (148.5, 105) ccw
  arc A390 (148.1008, 76.2528) -> (148.8992, 76.2528) centre (148.5, 105) ccw
  arc A391 (151.1079, 76.3685) -> (151.9019, 76.452) centre (148.5, 105) ccw
  arc A392 (154.0864, 76.798) -> (154.8674, 76.964) centre (148.5, 105) ccw
  arc A393 (157.0037, 77.5364) -> (157.7631, 77.7831) centre (148.5, 105) ccw
  arc A394 (159.8278, 78.5757) -> (160.5573, 78.9005) centre (148.5, 105) ccw
  arc A395 (162.5279, 79.9046) -> (163.2193, 80.3038) centre (148.5, 105) ccw
  arc A396 (165.0742, 81.5084) -> (165.7202, 81.9777) centre (148.5, 105) ccw
  arc A397 (167.439, 83.3695) -> (168.0323, 83.9038) centre (148.5, 105) ccw
  arc A398 (169.5962, 85.4677) -> (170.1305, 86.061) centre (148.5, 105) ccw
  arc A399 (171.5223, 87.7798) -> (171.9916, 88.4258) centre (148.5, 105) ccw
  arc A400 (173.1962, 90.2807) -> (173.5954, 90.9721) centre (148.5, 105) ccw
  arc A401 (174.5995, 92.9427) -> (174.9243, 93.6722) centre (148.5, 105) ccw
  arc A402 (175.7169, 95.7369) -> (175.9636, 96.4963) centre (148.5, 105) ccw
  arc A403 (176.536, 98.6326) -> (176.702, 99.4136) centre (148.5, 105) ccw
  arc A404 (177.048, 101.5981) -> (177.1315, 102.3921) centre (148.5, 105) ccw
  arc A405 (177.2472, 104.6008) -> (177.2472, 105.3992) centre (148.5, 105) ccw
  arc A406 (177.1315, 107.6079) -> (177.048, 108.4019) centre (148.5, 105) ccw
  arc A407 (176.702, 110.5864) -> (176.536, 111.3674) centre (148.5, 105) ccw
  arc A408 (175.9636, 113.5037) -> (175.7169, 114.2631) centre (148.5, 105) ccw
  arc A409 (174.9243, 116.3278) -> (174.5995, 117.0573) centre (148.5, 105) ccw
  arc A410 (173.5954, 119.0279) -> (173.1962, 119.7193) centre (148.5, 105) ccw
  arc A411 (171.9916, 121.5742) -> (171.5223, 122.2202) centre (148.5, 105) ccw
  arc A412 (170.1305, 123.939) -> (169.5962, 124.5323) centre (148.5, 105) ccw
  arc A413 (168.0323, 126.0962) -> (167.439, 126.6305) centre (148.5, 105) ccw
  arc A414 (165.7202, 128.0223) -> (165.0742, 128.4916) centre (148.5, 105) ccw
  arc A415 (163.2193, 129.6962) -> (162.5279, 130.0954) centre (148.5, 105) ccw
  arc A416 (160.5573, 131.0995) -> (159.8278, 131.4243) centre (148.5, 105) ccw
  arc A417 (157.7631, 132.2169) -> (157.0037, 132.4636) centre (148.5, 105) ccw
  arc A418 (154.8674, 133.036) -> (154.0864, 133.202) centre (148.5, 105) ccw
  arc A419 (151.9019, 133.548) -> (151.1079, 133.6315) centre (148.5, 105) ccw
  arc A420 (147.27, 135.9756) -> (146.4854, 135.9345) centre (148.5, 105) ccw
  arc A421 (144.0389, 135.6773) -> (143.2629, 135.5544) centre (148.5, 105) ccw
  arc A422 (140.8567, 135.043) -> (140.0978, 134.8396) centre (148.5, 105) ccw
  arc A423 (137.7582, 134.0794) -> (137.0248, 133.7979) centre (148.5, 105) ccw
  arc A424 (134.7774, 132.7973) -> (134.0774, 132.4406) centre (148.5, 105) ccw
  arc A425 (131.947, 131.2106) -> (131.2881, 130.7827) centre (148.5, 105) ccw
  arc A426 (129.2979, 129.3368) -> (128.6874, 128.8424) centre (148.5, 105) ccw
  arc A427 (126.8592, 127.1963) -> (126.3037, 126.6408) centre (148.5, 105) ccw
  arc A428 (124.6576, 124.8126) -> (124.1632, 124.2021) centre (148.5, 105) ccw
  arc A429 (122.7173, 122.2119) -> (122.2894, 121.553) centre (148.5, 105) ccw
  arc A430 (121.0594, 119.4226) -> (120.7027, 118.7226) centre (148.5, 105) ccw
  arc A431 (119.7021, 116.4752) -> (119.4206, 115.7418) centre (148.5, 105) ccw
  arc A432 (118.6604, 113.4022) -> (118.457, 112.6433) centre (148.5, 105) ccw
  arc A433 (117.9456, 110.2371) -> (117.8227, 109.4611) centre (148.5, 105) ccw
  arc A434 (117.5655, 107.0146) -> (117.5244, 106.23) centre (148.5, 105) ccw
  arc A435 (117.5244, 103.77) -> (117.5655, 102.9854) centre (148.5, 105) ccw
  arc A436 (117.8227, 100.5389) -> (117.9456, 99.7629) centre (148.5, 105) ccw
  arc A437 (118.457, 97.3567) -> (118.6604, 96.5978) centre (148.5, 105) ccw
  arc A438 (119.4206, 94.2582) -> (119.7021, 93.5248) centre (148.5, 105) ccw
  arc A439 (120.7027, 91.2774) -> (121.0594, 90.5774) centre (148.5, 105) ccw
  arc A440 (122.2894, 88.447) -> (122.7173, 87.7881) centre (148.5, 105) ccw
  arc A441 (124.1632, 85.7979) -> (124.6576, 85.1874) centre (148.5, 105) ccw
  arc A442 (126.3037, 83.3592) -> (126.8592, 82.8037) centre (148.5, 105) ccw
  arc A443 (128.6874, 81.1576) -> (129.2979, 80.6632) centre (148.5, 105) ccw
  arc A444 (131.2881, 79.2173) -> (131.947, 78.7894) centre (148.5, 105) ccw
  arc A445 (134.0774, 77.5594) -> (134.7774, 77.2027) centre (148.5, 105) ccw
  arc A446 (137.0248, 76.2021) -> (137.7582, 75.9206) centre (148.5, 105) ccw
  arc A447 (140.0978, 75.1604) -> (140.8567, 74.957) centre (148.5, 105) ccw
  arc A448 (143.2629, 74.4456) -> (144.0389, 74.3227) centre (148.5, 105) ccw
  arc A449 (146.4854, 74.0655) -> (147.27, 74.0244) centre (148.5, 105) ccw
  arc A450 (149.73, 74.0244) -> (150.5146, 74.0655) centre (148.5, 105) ccw
  arc A451 (152.9611, 74.3227) -> (153.7371, 74.4456) centre (148.5, 105) ccw
  arc A452 (156.1433, 74.957) -> (156.9022, 75.1604) centre (148.5, 105) ccw
  arc A453 (159.2418, 75.9206) -> (159.9752, 76.2021) centre (148.5, 105) ccw
  arc A454 (162.2226, 77.2027) -> (162.9226, 77.5594) centre (148.5, 105) ccw
  arc A455 (165.053, 78.7894) -> (165.7119, 79.2173) centre (148.5, 105) ccw
  arc A456 (167.7021, 80.6632) -> (168.3126, 81.1576) centre (148.5, 105) ccw
  arc A457 (170.1408, 82.8037) -> (170.6963, 83.3592) centre (148.5, 105) ccw
  arc A458 (172.3424, 85.1874) -> (172.8368, 85.7979) centre (148.5, 105) ccw
  arc A459 (174.2827, 87.7881) -> (174.7106, 88.447) centre (148.5, 105) ccw
  arc A460 (175.9406, 90.5774) -> (176.2973, 91.2774) centre (148.5, 105) ccw
  arc A461 (177.2979, 93.5248) -> (177.5794, 94.2582) centre (148.5, 105) ccw
  arc A462 (178.3396, 96.5978) -> (178.543, 97.3567) centre (148.5, 105) ccw
  arc A463 (179.0544, 99.7629) -> (179.1773, 100.5389) centre (148.5, 105) ccw
  arc A464 (179.4345, 102.9854) -> (179.4756, 103.77) centre (148.5, 105) ccw
  arc A465 (179.4756, 106.23) -> (179.4345, 107.0146) centre (148.5, 105) ccw
  arc A466 (179.1773, 109.4611) -> (179.0544, 110.2371) centre (148.5, 105) ccw
  arc A467 (178.543, 112.6433) -> (178.3396, 113.4022) centre (148.5, 105) ccw
  arc A468 (177.5794, 115.7418) -> (177.2979, 116.4752) centre (148.5, 105) ccw
  arc A469 (176.2973, 118.7226) -> (175.9406, 119.4226) centre (148.5, 105) ccw
  arc A470 (174.7106, 121.553) -> (174.2827, 122.2119) centre (148.5, 105) ccw
  arc A471 (172.8368, 124.2021) -> (172.3424, 124.8126) centre (148.5, 105) ccw
  arc A472 (170.6963, 126.6408) -> (170.1408, 127.1963) centre (148.5, 105) ccw
  arc A473 (168.3126, 128.8424) -> (167.7021, 129.3368) centre (148.5, 105) ccw
  arc A474 (165.7119, 130.7827) -> (165.053, 131.2106) centre (148.5, 105) ccw
  arc A475 (162.9226, 132.4406) -> (162.2226, 132.7973) centre (148.5, 105) ccw
  arc A476 (159.9752, 133.7979) -> (159.2418, 134.0794) centre (148.5, 105) ccw
  arc A477 (156.9022, 134.8396) -> (156.1433, 135.043) centre (148.5, 105) ccw
  arc A478 (153.7371, 135.5544) -> (152.9611, 135.6773) centre (148.5, 105) ccw
  arc A479 (150.5146, 135.9345) -> (149.73, 135.9756) centre (148.5, 105) ccw
  line L0 (115.5, 105) -> (181.5, 105) construction
  line L1 (148.5, 72) -> (148.5, 138) construction
  line L2 (199.5, 136) -> (269.5, 136)
  line L3 (199.5, 128) -> (269.5, 128)
  line L4 (199.5, 120) -> (269.5, 120)
  line L5 (199.5, 112) -> (269.5, 112)
  line L6 (199.5, 104) -> (269.5, 104)
  line L7 (199.5, 96) -> (269.5, 96)
  line L8 (199.5, 88) -> (269.5, 88)
  line L9 (199.5, 80) -> (269.5, 80)
  line L10 (199.5, 72) -> (269.5, 72)
  line L11 (199.5, 64) -> (269.5, 64)
  line L12 (199.5, 56) -> (269.5, 56)
  line L13 (199.5, 48) -> (269.5, 48)
  line L14 (199.5, 40) -> (269.5, 40)
  line L15 (199.5, 136) -> (199.5, 40)
  line L16 (269.5, 136) -> (269.5, 40)
  line L17 (234.5, 128) -> (234.5, 40)
  circle A480 centre (148.5, 105) radius 5.025 construction
  circle A481 centre (148.5, 105) radius 8.025
  circle A482 centre (148.5, 105) radius 24.75
  line L18 (145.5, 72) -> (145.5, 138) construction
  line L19 (151.5, 72) -> (151.5, 138) construction
  line L20 (115.5, 108) -> (181.5, 108) construction
  line L21 (115.5, 102) -> (181.5, 102) construction
  line L22 (145.5, 129.5675) -> (144.2584, 111.8125)
  line L23 (151.5, 129.5675) -> (152.7416, 111.8125)
  line L24 (123.9325, 102) -> (141.6875, 100.7584)
  line L25 (123.9325, 108) -> (141.6875, 109.2416)
  line L26 (151.5, 80.4325) -> (152.7416, 98.1875)
  line L27 (145.5, 80.4325) -> (144.2584, 98.1875)
  line L28 (173.0675, 108) -> (155.3125, 109.2416)
  line L29 (173.0675, 102) -> (155.3125, 100.7584)
  circle A483 centre (-2.1213, 2.1213) radius 1.25 construction
  circle A484 centre (2.1213, -2.1213) radius 1.25 construction
  circle A485 centre (0, 0) radius 6 construction
  circle A486 centre (0, 0) radius 9
  circle A487 centre (-12.7279, -12.7279) radius 1.25 construction
  circle A488 centre (0, 0) radius 5.2 construction
  line L30 (0, 0) -> (-3.677, 3.677) construction
  line L31 (-3.677, 3.677) -> (1.3459, 5.0228) construction
  line L32 (1.3459, 5.0228) -> (5.0228, 1.3459) construction
  line L33 (5.0228, 1.3459) -> (3.677, -3.677) construction
  line L34 (3.677, -3.677) -> (-1.3459, -5.0228) construction
  line L35 (-1.3459, -5.0228) -> (-5.0228, -1.3459) construction
  line L36 (-5.0228, -1.3459) -> (-3.677, 3.677) construction
  arc A489 (-2.6052, 3.9641) -> (-3.677, 3.677) centre (-2.8924, 2.8924) ccw
  arc A490 (-3.677, 3.677) -> (-3.9641, 2.6052) centre (-2.8924, 2.8924) ccw
  arc A491 (-4.7356, -0.2741) -> (-5.0228, -1.3459) centre (-3.951, -1.0587) ccw
  arc A492 (-5.0228, -1.3459) -> (-4.2382, -2.1305) centre (-3.951, -1.0587) ccw
  arc A493 (-2.1305, -4.2382) -> (-1.3459, -5.0228) centre (-1.0587, -3.951) ccw
  arc A494 (-1.3459, -5.0228) -> (-0.2741, -4.7356) centre (-1.0587, -3.951) ccw
  arc A495 (2.6052, -3.9641) -> (3.677, -3.677) centre (2.8924, -2.8924) ccw
  arc A496 (3.677, -3.677) -> (3.9641, -2.6052) centre (2.8924, -2.8924) ccw
  arc A497 (4.7356, 0.2741) -> (5.0228, 1.3459) centre (3.951, 1.0587) ccw
  arc A498 (5.0228, 1.3459) -> (4.2382, 2.1305) centre (3.951, 1.0587) ccw
  arc A499 (2.1305, 4.2382) -> (1.3459, 5.0228) centre (1.0587, 3.951) ccw
  arc A500 (1.3459, 5.0228) -> (0.2741, 4.7356) centre (1.0587, 3.951) ccw
  arc A501 (-2.6052, 3.9641) -> (0.2741, 4.7356) centre (-1.8337, 6.8434) ccw
  arc A502 (-4.7356, -0.2741) -> (-3.9641, 2.6052) centre (-6.8434, 1.8337) ccw
  arc A503 (-2.1305, -4.2382) -> (-4.2382, -2.1305) centre (-5.0097, -5.0097) ccw
  arc A504 (2.6052, -3.9641) -> (-0.2741, -4.7356) centre (1.8337, -6.8434) ccw
  arc A505 (4.7356, 0.2741) -> (3.9641, -2.6052) centre (6.8434, -1.8337) ccw
  arc A506 (2.1305, 4.2382) -> (4.2382, 2.1305) centre (5.0097, 5.0097) ccw
  circle A507 centre (-12.7279, -12.7279) radius 6
  circle A508 centre (-12.7279, -12.7279) radius 9
  circle A509 centre (-12.7279, -12.7279) radius 1.5
  circle A510 centre (-12.7279, -12.7279) radius 5.2 construction
  line L37 (-12.7279, -12.7279) -> (-12.7279, -7.5279) construction
  line L38 (-12.7279, -7.5279) -> (-8.2246, -10.1279) construction
  line L39 (-8.2246, -10.1279) -> (-8.2246, -15.3279) construction
  line L40 (-8.2246, -15.3279) -> (-12.7279, -17.9279) construction
  line L41 (-12.7279, -17.9279) -> (-17.2313, -15.3279) construction
  line L42 (-17.2313, -15.3279) -> (-17.2313, -10.1279) construction
  line L43 (-17.2313, -10.1279) -> (-12.7279, -7.5279) construction
  arc A511 (-11.767, -8.0827) -> (-12.7279, -7.5279) centre (-12.7279, -8.6375) ccw
  arc A512 (-12.7279, -7.5279) -> (-13.6889, -8.0827) centre (-12.7279, -8.6375) ccw
  arc A513 (-16.2703, -9.5731) -> (-17.2313, -10.1279) centre (-16.2703, -10.6827) ccw
  arc A514 (-17.2313, -10.1279) -> (-17.2313, -11.2375) centre (-16.2703, -10.6827) ccw
  arc A515 (-17.2313, -14.2183) -> (-17.2313, -15.3279) centre (-16.2703, -14.7731) ccw
  arc A516 (-17.2313, -15.3279) -> (-16.2703, -15.8827) centre (-16.2703, -14.7731) ccw
  arc A517 (-13.6889, -17.3731) -> (-12.7279, -17.9279) centre (-12.7279, -16.8183) ccw
  arc A518 (-12.7279, -17.9279) -> (-11.767, -17.3731) centre (-12.7279, -16.8183) ccw
  arc A519 (-9.1855, -15.8827) -> (-8.2246, -15.3279) centre (-9.1855, -14.7731) ccw
  arc A520 (-8.2246, -15.3279) -> (-8.2246, -14.2183) centre (-9.1855, -14.7731) ccw
  arc A521 (-8.2246, -11.2375) -> (-8.2246, -10.1279) centre (-9.1855, -10.6827) ccw
  arc A522 (-8.2246, -10.1279) -> (-9.1855, -9.5731) centre (-9.1855, -10.6827) ccw
  arc A523 (-11.767, -8.0827) -> (-9.1855, -9.5731) centre (-9.1855, -6.5923) ccw
  arc A524 (-16.2703, -9.5731) -> (-13.6889, -8.0827) centre (-16.2703, -6.5923) ccw
  arc A525 (-17.2313, -14.2183) -> (-17.2313, -11.2375) centre (-19.8127, -12.7279) ccw
  arc A526 (-13.6889, -17.3731) -> (-16.2703, -15.8827) centre (-16.2703, -18.8635) ccw
  arc A527 (-9.1855, -15.8827) -> (-11.767, -17.3731) centre (-9.1855, -18.8635) ccw
  arc A528 (-8.2246, -11.2375) -> (-8.2246, -14.2183) centre (-5.6431, -12.7279) ccw
  arc A529 (-1.682, 8.8414) -> (-21.5694, -11.0459) centre (2.9902, -15.7181) ccw
  arc A530 (-11.0459, -21.5694) -> (8.8414, -1.682) centre (-15.7181, 2.9902) ccw
  circle A531 centre (0, 0) radius 1.25
  circle A532 centre (148.5, 105) radius 5.2 construction
  line L44 (148.5, 105) -> (148.5, 110.2) construction
  line L45 (148.5, 110.2) -> (153.0033, 107.6) construction
  line L46 (153.0033, 107.6) -> (153.0033, 102.4) construction
  line L47 (153.0033, 102.4) -> (148.5, 99.8) construction
  line L48 (148.5, 99.8) -> (143.9967, 102.4) construction
  line L49 (143.9967, 102.4) -> (143.9967, 107.6) construction
  line L50 (143.9967, 107.6) -> (148.5, 110.2) construction
  arc A533 (149.4609, 109.6452) -> (147.5391, 109.6452) centre (148.5, 109.0904) ccw
  arc A534 (144.9576, 108.1548) -> (143.9967, 106.4904) centre (144.9576, 107.0452) ccw
  arc A535 (143.9967, 103.5096) -> (144.9576, 101.8452) centre (144.9576, 102.9548) ccw
  arc A536 (147.5391, 100.3548) -> (149.4609, 100.3548) centre (148.5, 100.9096) ccw
  arc A537 (152.0424, 101.8452) -> (153.0033, 103.5096) centre (152.0424, 102.9548) ccw
  arc A538 (153.0033, 106.4904) -> (152.0424, 108.1548) centre (152.0424, 107.0452) ccw
  arc A539 (144.9576, 108.1548) -> (147.5391, 109.6452) centre (144.9576, 111.1356) ccw
  arc A540 (143.9967, 103.5096) -> (143.9967, 106.4904) centre (141.4152, 105) ccw
  arc A541 (147.5391, 100.3548) -> (144.9576, 101.8452) centre (144.9576, 98.8644) ccw
  arc A542 (152.0424, 101.8452) -> (149.4609, 100.3548) centre (152.0424, 98.8644) ccw
  arc A543 (153.0033, 106.4904) -> (153.0033, 103.5096) centre (155.5848, 105) ccw
  arc A544 (149.4609, 109.6452) -> (152.0424, 108.1548) centre (152.0424, 111.1356) ccw
  circle A545 centre (148.5, 105) radius 1.5
  point P0 (205.5, 130)
  point P1 (208, 122)
  point P2 (208, 114)
  point P3 (205.5, 106)
  point P4 (208, 98)
  point P5 (203, 90)
  point P6 (205.5, 82)
  point P7 (205.5, 74)
  point P8 (205.5, 66)
  point P9 (208, 58)
  point P10 (208, 50)
  point P11 (205.5, 42)
  point P12 (235.5, 122)
  point P13 (250.5, 114)
  point P14 (251.75, 106)
  point P15 (248, 98)
  point P16 (250.5, 90)
  point P17 (244.25, 82)
  point P18 (250.5, 74)
  point P19 (248, 66)
  point P20 (245.5, 58)
  point P21 (253, 50)
  point P22 (253, 42)
  point P23 (149.5, 151.5)
  point P24 (149.5, 145.5)
  point P25 (165.6875, 151.5)
  point P26 (167.8125, 145.5)
  point P27 (155.3125, 109.2416)
  point P28 (144.2584, 98.1875)
  point P29 (143.9967, 107.6)
  point P30 (148.5, 99.8)
  point P31 (153.0033, 102.4)
  point P32 (153.0033, 107.6)
  point P33 (143.9967, 106.4904)
  point P34 (143.9967, 103.5096)
  point P35 (144.9576, 101.8452)
  point P36 (149.4609, 100.3548)
  point P37 (152.0424, 101.8452)
  point P38 (153.0033, 103.5096)
  point P39 (152.0424, 108.1548)
  dimension "d0" = 10.05
  dimension "d7" = 3
  dimension "d8" = 4
  dimension "d9" = 3
  dimension "d10" = 3
  dimension "d11" = 3
  dimension "d12" = 3
  dimension "d13" = 4
  dimension "d14" = 4
  dimension "d17" = 360
  dimension "d38" = 12
  dimension "d39" = 18
  dimension "d41" = 360